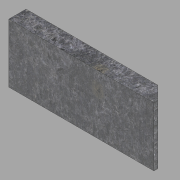
# Autodesk Inventor part: 1-80
Saved by Autodesk Inventor 2022.2 (Build 262287000, 287)
## iProperties
Created: 2021-12-23
Part Number: 1-80
Material: Granite, Cut, Polished
Document SubType Name: Modeling
Designer: awelt
Density: 2.7 g/cm^3
Appearance: Kasota SN sapphire
Mass: 13763.4 g
Surface Area: 2548.22 cm^2
Volume: 5097.55 cm^3
Author: awelt
Revision Number: 2
Autodesk Inventor part; units mm, degrees
ref_plane "YZ Plane" through (0, 0, 0) normal (1, 0, 0) x (0, 1, 0)
ref_plane "XZ Plane" through (0, 0, 0) normal (0, 1, 0) x (-1, 0, 0)
ref_plane "XY Plane" through (0, 0, 0) normal (0, 0, 1) x (1, 0, 0)
sketch "Sketch1" plane through (0, 0, 0) normal (1, 0, 0) x (0, 1, 0)
  line L0 (0, 0) -> (57.15, 0)
  line L1 (57.15, 0) -> (57.15, 193.675)
  line L2 (57.15, 193.675) -> (0, 193.675)
  line L3 (0, 193.675) -> (0, 0)
  dimension "d0" = 57.15
  dimension "d1" = 193.675
  constraints: 8 end point, 2 parallel, 1 horizontal, 1 perpendicular
  measures "d0" distance of L2.end L1.end
  measures "d1" distance of L1.end L0.end
extrude "Extrusion1" add sketch "Sketch1" along normal blind 477.8375
sketch "Sketch3" plane through (0, 0, 0) normal (0, 0, -1) x (-1, 0, 0)
  line L0 (-477.8375, 0) -> (-397.0152, 0) construction
  line L1 (-477.8375, 57.15) -> (-477.8375, 0)
  line L2 (0, 0) -> (-477.8375, 0) projected
  line L3 (-477.8375, 57.15) -> (-420.6875, 0)
  line L4 (-477.8375, 57.15) -> (-477.8375, 0) projected
  line L5 (-477.8375, 0) -> (-420.6875, 0)
  constraints: 8 end point, 1 collinear, 1 horizontal, 1 point on line
extrude "Extrusion3" cut sketch "Sketch3" against normal up to surface (193.675 mm away)
thicken "Thicken1" operation add thickness 3.175 both sides no extend neighbours yes toward (-0.7071068, 0.7071068, 0) faces at (458.7875, 38.1, 129.1167)
sketch "Sketch4" plane through (0, 0, 0) normal (0, 0, -1) x (-1, 0, 0)
  line L0 (0, 57.15) -> (-473.3474, 57.15) projected
  line L1 (-460.6474, 57.15) -> (-460.6474, 44.45)
  line L2 (-473.3474, 57.15) -> (-416.1974, 0) projected
  line L3 (-473.3474, 57.15) -> (-460.6474, 57.15)
  line L4 (-460.6474, 44.45) -> (-473.3474, 57.15)
  point P0 (0, 0)
  dimension "d17" = 12.7
  constraints: 6 end point, 2 point on line, 1 perpendicular, 1 vertical
  measures "d17" distance of L1.start L1.end
extrude "Extrusion4" cut sketch "Sketch4" against normal blind 193.675
sketch "Sketch6" plane through (0, 0, 0) normal (-1, 0, 0) x (0, 0, 1)
  line L0 (0, 57.15) -> (193.675, 57.15) projected
  line L1 (0, 0) -> (193.675, 0)
  line L2 (193.675, 0) -> (193.675, 57.15)
  line L3 (193.675, 57.15) -> (0, 57.15)
  line L4 (0, 57.15) -> (0, 0)
  constraints: 8 end point, 2 parallel, 1 horizontal, 1 perpendicular
extrude "Extrusion5" add sketch "Sketch6" along normal blind 17.1831
body "Solid1"
